Autodesk Inventor part; units mm, degrees
(part 3 of 4)
  spline S47 degree 5 poles (5.1648, 1.4192) (5.1666, 1.4197) (5.1702, 1.4206) (5.1756, 1.4219) (5.1829, 1.4234) (5.1921, 1.425) (5.2013, 1.4263) (5.2105, 1.4276) (5.2198, 1.4287) (5.2291, 1.4298) (5.2384, 1.4308) (5.2477, 1.4317) (5.257, 1.4326) (5.2664, 1.4333) (5.2758, 1.434) (5.2852, 1.4345) (5.2947, 1.435) (5.3041, 1.4354) (5.3136, 1.4357) (5.3231, 1.436) (5.3326, 1.4362) (5.3421, 1.4363) (5.3517, 1.4364) (5.3612, 1.4364) (5.3708, 1.4363) (5.3803, 1.4362) (5.3899, 1.436) (5.3995, 1.4357) (5.4091, 1.4354) (5.4188, 1.4351) (5.4284, 1.4347) (5.4381, 1.4342) (5.4477, 1.4337) (5.4574, 1.4331) (5.4671, 1.4324) (5.4768, 1.4317) (5.4865, 1.431) (5.4962, 1.4302) (5.5059, 1.4294) (5.5156, 1.4285) (5.5254, 1.4275) (5.5351, 1.4265) (5.5449, 1.4255) (5.5546, 1.4244) (5.5644, 1.4232) (5.5742, 1.422) (5.584, 1.4208) (5.5938, 1.4195) (5.6036, 1.4182) (5.6134, 1.4168) (5.6232, 1.4154) (5.633, 1.4139) (5.6429, 1.4124) (5.6527, 1.4108) (5.6626, 1.4092) (5.6724, 1.4075) (5.6823, 1.4058) (5.6922, 1.4041) (5.702, 1.4023) (5.7119, 1.4005) (5.7218, 1.3986) (5.7317, 1.3967) (5.7416, 1.3947) (5.7515, 1.3927) (5.7614, 1.3907) (5.7713, 1.3886) (5.7812, 1.3865) (5.7912, 1.3843) (5.8051, 1.3812) (5.817, 1.3785) (5.8269, 1.3761) (5.8349, 1.3742) (5.8408, 1.3728) knots 0 0 0 0 0 0 0.014286 0.028571 0.042857 0.057143 0.071429 0.085714 0.1 0.114286 0.128571 0.142857 0.157143 0.171429 0.185714 0.2 0.214286 0.228571 0.242857 0.257143 0.271429 0.285714 0.3 0.314286 0.328571 0.342857 0.357143 0.371429 0.385714 0.4 0.414286 0.428571 0.442857 0.457143 0.471429 0.485714 0.5 0.514286 0.528571 0.542857 0.557143 0.571429 0.585714 0.6 0.614286 0.628571 0.642857 0.657143 0.671429 0.685714 0.7 0.714286 0.728571 0.742857 0.757143 0.771429 0.785714 0.8 0.814286 0.828571 0.842857 0.857143 0.871429 0.885714 0.9 0.914286 0.928571 0.942857 0.957143 1 1 1 1 1 1
  line L47 (5.1, 1.4019) -> (5.1648, 1.4192)
  arc A48 (5.1, 1.4019) -> (5.0177, 1.6729) centre (0, 0) ccw
  line L48 (5.0177, 1.6729) -> (5.0811, 1.6946)
  spline S48 degree 5 poles (5.0811, 1.6946) (5.0829, 1.6952) (5.0864, 1.6964) (5.0916, 1.6984) (5.0985, 1.7012) (5.107, 1.705) (5.1154, 1.709) (5.1237, 1.7131) (5.1321, 1.7173) (5.1404, 1.7216) (5.1487, 1.7259) (5.157, 1.7303) (5.1652, 1.7348) (5.1734, 1.7394) (5.1816, 1.7441) (5.1897, 1.7489) (5.1978, 1.7537) (5.2059, 1.7587) (5.2139, 1.7637) (5.222, 1.7687) (5.23, 1.7739) (5.238, 1.7791) (5.2459, 1.7843) (5.2539, 1.7896) (5.2618, 1.795) (5.2697, 1.8004) (5.2775, 1.8059) (5.2854, 1.8115) (5.2932, 1.8171) (5.301, 1.8227) (5.3087, 1.8284) (5.3165, 1.8342) (5.3242, 1.84) (5.3319, 1.8459) (5.3396, 1.8518) (5.3473, 1.8578) (5.3549, 1.8638) (5.3626, 1.8698) (5.3702, 1.8759) (5.3778, 1.8821) (5.3853, 1.8883) (5.3929, 1.8946) (5.4004, 1.9009) (5.4079, 1.9072) (5.4154, 1.9136) (5.4228, 1.92) (5.4303, 1.9265) (5.4377, 1.933) (5.4451, 1.9396) (5.4525, 1.9462) (5.4599, 1.9529) (5.4672, 1.9595) (5.4745, 1.9663) (5.4819, 1.9731) (5.4891, 1.9799) (5.4964, 1.9867) (5.5037, 1.9936) (5.5109, 2.0006) (5.5181, 2.0075) (5.5253, 2.0146) (5.5325, 2.0216) (5.5396, 2.0287) (5.5467, 2.0359) (5.5539, 2.043) (5.561, 2.0502) (5.568, 2.0575) (5.5751, 2.0648) (5.5821, 2.0721) (5.5919, 2.0824) (5.6003, 2.0913) (5.6073, 2.0988) (5.6129, 2.1048) (5.617, 2.1093) knots 0 0 0 0 0 0 0.014286 0.028571 0.042857 0.057143 0.071429 0.085714 0.1 0.114286 0.128571 0.142857 0.157143 0.171429 0.185714 0.2 0.214286 0.228571 0.242857 0.257143 0.271429 0.285714 0.3 0.314286 0.328571 0.342857 0.357143 0.371429 0.385714 0.4 0.414286 0.428571 0.442857 0.457143 0.471429 0.485714 0.5 0.514286 0.528571 0.542857 0.557143 0.571429 0.585714 0.6 0.614286 0.628571 0.642857 0.657143 0.671429 0.685714 0.7 0.714286 0.728571 0.742857 0.757143 0.771429 0.785714 0.8 0.814286 0.828571 0.842857 0.857143 0.871429 0.885714 0.9 0.914286 0.928571 0.942857 0.957143 1 1 1 1 1 1
  arc A49 (5.617, 2.1093) -> (5.5352, 2.3155) centre (0, 0) ccw
  spline S49 degree 5 poles (4.8608, 2.25) (4.8625, 2.2507) (4.8659, 2.2522) (4.871, 2.2544) (4.8779, 2.2571) (4.8867, 2.2601) (4.8956, 2.263) (4.9045, 2.2657) (4.9134, 2.2684) (4.9224, 2.2709) (4.9314, 2.2735) (4.9405, 2.2759) (4.9496, 2.2783) (4.9587, 2.2806) (4.9678, 2.2828) (4.977, 2.2849) (4.9863, 2.2869) (4.9955, 2.2888) (5.0048, 2.2907) (5.0142, 2.2925) (5.0235, 2.2943) (5.0329, 2.296) (5.0422, 2.2976) (5.0517, 2.2992) (5.0611, 2.3007) (5.0706, 2.3022) (5.0801, 2.3036) (5.0896, 2.3049) (5.0991, 2.3062) (5.1087, 2.3074) (5.1182, 2.3086) (5.1278, 2.3097) (5.1374, 2.3108) (5.1471, 2.3118) (5.1567, 2.3128) (5.1664, 2.3137) (5.1761, 2.3145) (5.1858, 2.3153) (5.1955, 2.3161) (5.2053, 2.3168) (5.215, 2.3175) (5.2248, 2.3181) (5.2346, 2.3187) (5.2444, 2.3192) (5.2543, 2.3197) (5.2641, 2.3201) (5.274, 2.3205) (5.2838, 2.3209) (5.2937, 2.3212) (5.3036, 2.3214) (5.3136, 2.3216) (5.3235, 2.3218) (5.3335, 2.3219) (5.3434, 2.322) (5.3534, 2.322) (5.3634, 2.322) (5.3734, 2.3219) (5.3834, 2.3219) (5.3934, 2.3217) (5.4035, 2.3215) (5.4136, 2.3213) (5.4236, 2.3211) (5.4337, 2.3207) (5.4438, 2.3204) (5.4539, 2.32) (5.464, 2.3196) (5.4742, 2.3191) (5.4843, 2.3186) (5.4985, 2.3178) (5.5107, 2.3171) (5.5209, 2.3165) (5.5291, 2.3159) (5.5352, 2.3155) knots 0 0 0 0 0 0 0.014286 0.028571 0.042857 0.057143 0.071429 0.085714 0.1 0.114286 0.128571 0.142857 0.157143 0.171429 0.185714 0.2 0.214286 0.228571 0.242857 0.257143 0.271429 0.285714 0.3 0.314286 0.328571 0.342857 0.357143 0.371429 0.385714 0.4 0.414286 0.428571 0.442857 0.457143 0.471429 0.485714 0.5 0.514286 0.528571 0.542857 0.557143 0.571429 0.585714 0.6 0.614286 0.628571 0.642857 0.657143 0.671429 0.685714 0.7 0.714286 0.728571 0.742857 0.757143 0.771429 0.785714 0.8 0.814286 0.828571 0.842857 0.857143 0.871429 0.885714 0.9 0.914286 0.928571 0.942857 0.957143 1 1 1 1 1 1
  line L49 (4.7997, 2.2222) -> (4.8608, 2.25)
  arc A50 (4.7997, 2.2222) -> (4.6739, 2.476) centre (0, 0) ccw
  line L50 (4.6739, 2.476) -> (4.7329, 2.5078)
  spline S50 degree 5 poles (4.7329, 2.5078) (4.7345, 2.5087) (4.7378, 2.5105) (4.7426, 2.5133) (4.7489, 2.5172) (4.7567, 2.5223) (4.7643, 2.5276) (4.7719, 2.533) (4.7794, 2.5386) (4.7869, 2.5442) (4.7944, 2.5498) (4.8018, 2.5555) (4.8092, 2.5613) (4.8166, 2.5672) (4.8238, 2.5732) (4.8311, 2.5792) (4.8383, 2.5854) (4.8454, 2.5916) (4.8525, 2.5978) (4.8596, 2.6041) (4.8667, 2.6105) (4.8737, 2.6169) (4.8807, 2.6234) (4.8876, 2.63) (4.8946, 2.6366) (4.9014, 2.6432) (4.9083, 2.6499) (4.9151, 2.6567) (4.9219, 2.6635) (4.9287, 2.6704) (4.9354, 2.6773) (4.9421, 2.6842) (4.9488, 2.6912) (4.9554, 2.6983) (4.962, 2.7054) (4.9686, 2.7125) (4.9751, 2.7197) (4.9817, 2.727) (4.9882, 2.7343) (4.9946, 2.7416) (5.0011, 2.749) (5.0075, 2.7564) (5.0139, 2.7638) (5.0202, 2.7713) (5.0266, 2.7788) (5.0329, 2.7864) (5.0391, 2.794) (5.0454, 2.8017) (5.0516, 2.8094) (5.0578, 2.8171) (5.064, 2.8249) (5.0701, 2.8327) (5.0762, 2.8405) (5.0823, 2.8484) (5.0884, 2.8564) (5.0944, 2.8643) (5.1005, 2.8723) (5.1064, 2.8803) (5.1124, 2.8884) (5.1183, 2.8965) (5.1243, 2.9047) (5.1301, 2.9128) (5.136, 2.9211) (5.1418, 2.9293) (5.1477, 2.9376) (5.1534, 2.9459) (5.1592, 2.9542) (5.1649, 2.9626) (5.1729, 2.9744) (5.1797, 2.9846) (5.1854, 2.9931) (5.1899, 2.9999) (5.1932, 3.0051) knots 0 0 0 0 0 0 0.014286 0.028571 0.042857 0.057143 0.071429 0.085714 0.1 0.114286 0.128571 0.142857 0.157143 0.171429 0.185714 0.2 0.214286 0.228571 0.242857 0.257143 0.271429 0.285714 0.3 0.314286 0.328571 0.342857 0.357143 0.371429 0.385714 0.4 0.414286 0.428571 0.442857 0.457143 0.471429 0.485714 0.5 0.514286 0.528571 0.542857 0.557143 0.571429 0.585714 0.6 0.614286 0.628571 0.642857 0.657143 0.671429 0.685714 0.7 0.714286 0.728571 0.742857 0.757143 0.771429 0.785714 0.8 0.814286 0.828571 0.842857 0.857143 0.871429 0.885714 0.9 0.914286 0.928571 0.942857 0.957143 1 1 1 1 1 1
  arc A51 (5.1932, 3.0051) -> (5.0786, 3.1949) centre (0, 0) ccw
  spline S51 degree 5 poles (4.4241, 3.0193) (4.4257, 3.0204) (4.4288, 3.0224) (4.4335, 3.0254) (4.4399, 3.0292) (4.4481, 3.0336) (4.4563, 3.0379) (4.4647, 3.0421) (4.473, 3.0461) (4.4815, 3.0502) (4.49, 3.0542) (4.4985, 3.0581) (4.507, 3.0619) (4.5157, 3.0657) (4.5244, 3.0693) (4.5331, 3.0729) (4.5419, 3.0764) (4.5507, 3.0799) (4.5595, 3.0832) (4.5684, 3.0866) (4.5773, 3.0898) (4.5863, 3.0931) (4.5953, 3.0962) (4.6043, 3.0993) (4.6134, 3.1024) (4.6225, 3.1054) (4.6316, 3.1083) (4.6408, 3.1112) (4.65, 3.114) (4.6592, 3.1168) (4.6684, 3.1195) (4.6777, 3.1222) (4.687, 3.1248) (4.6964, 3.1274) (4.7057, 3.13) (4.7151, 3.1325) (4.7245, 3.1349) (4.734, 3.1373) (4.7435, 3.1397) (4.753, 3.142) (4.7625, 3.1442) (4.772, 3.1465) (4.7816, 3.1486) (4.7912, 3.1508) (4.8008, 3.1529) (4.8104, 3.1549) (4.8201, 3.1569) (4.8298, 3.1589) (4.8395, 3.1608) (4.8492, 3.1627) (4.859, 3.1645) (4.8687, 3.1663) (4.8785, 3.1681) (4.8884, 3.1698) (4.8982, 3.1715) (4.9081, 3.1731) (4.9179, 3.1747) (4.9278, 3.1763) (4.9377, 3.1778) (4.9477, 3.1793) (4.9576, 3.1807) (4.9676, 3.1821) (4.9776, 3.1835) (4.9876, 3.1848) (4.9977, 3.1861) (5.0077, 3.1873) (5.0178, 3.1885) (5.0279, 3.1897) (5.042, 3.1913) (5.0542, 3.1926) (5.0644, 3.1936) (5.0725, 3.1944) (5.0786, 3.1949) knots 0 0 0 0 0 0 0.014286 0.028571 0.042857 0.057143 0.071429 0.085714 0.1 0.114286 0.128571 0.142857 0.157143 0.171429 0.185714 0.2 0.214286 0.228571 0.242857 0.257143 0.271429 0.285714 0.3 0.314286 0.328571 0.342857 0.357143 0.371429 0.385714 0.4 0.414286 0.428571 0.442857 0.457143 0.471429 0.485714 0.5 0.514286 0.528571 0.542857 0.557143 0.571429 0.585714 0.6 0.614286 0.628571 0.642857 0.657143 0.671429 0.685714 0.7 0.714286 0.728571 0.742857 0.757143 0.771429 0.785714 0.8 0.814286 0.828571 0.842857 0.857143 0.871429 0.885714 0.9 0.914286 0.928571 0.942857 0.957143 1 1 1 1 1 1
  line L51 (4.3685, 2.9819) -> (4.4241, 3.0193)
  arc A52 (4.3685, 2.9819) -> (4.2026, 3.2115) centre (0, 0) ccw
  line L52 (4.2026, 3.2115) -> (4.2556, 3.2526)
  spline S52 degree 5 poles (4.2556, 3.2526) (4.257, 3.2538) (4.26, 3.2561) (4.2643, 3.2596) (4.2699, 3.2645) (4.2767, 3.2708) (4.2833, 3.2773) (4.2899, 3.2839) (4.2964, 3.2906) (4.3029, 3.2974) (4.3093, 3.3042) (4.3157, 3.311) (4.3221, 3.3179) (4.3283, 3.325) (4.3345, 3.332) (4.3407, 3.3392) (4.3467, 3.3464) (4.3528, 3.3537) (4.3588, 3.3611) (4.3647, 3.3685) (4.3706, 3.3759) (4.3765, 3.3834) (4.3823, 3.391) (4.3881, 3.3986) (4.3938, 3.4062) (4.3995, 3.4139) (4.4052, 3.4217) (4.4108, 3.4295) (4.4164, 3.4373) (4.4219, 3.4452) (4.4274, 3.4531) (4.4329, 3.4611) (4.4383, 3.4691) (4.4437, 3.4771) (4.449, 3.4852) (4.4544, 3.4934) (4.4596, 3.5015) (4.4649, 3.5097) (4.4701, 3.518) (4.4753, 3.5263) (4.4804, 3.5346) (4.4855, 3.543) (4.4906, 3.5514) (4.4956, 3.5598) (4.5006, 3.5683) (4.5056, 3.5768) (4.5105, 3.5853) (4.5154, 3.5939) (4.5203, 3.6025) (4.5251, 3.6112) (4.53, 3.6199) (4.5347, 3.6286) (4.5395, 3.6373) (4.5442, 3.6461) (4.5489, 3.6549) (4.5535, 3.6638) (4.5581, 3.6726) (4.5627, 3.6816) (4.5673, 3.6905) (4.5718, 3.6995) (4.5763, 3.7085) (4.5807, 3.7175) (4.5852, 3.7266) (4.5896, 3.7357) (4.5939, 3.7448) (4.5983, 3.7539) (4.6026, 3.7631) (4.6069, 3.7723) (4.6128, 3.7853) (4.6178, 3.7964) (4.622, 3.8058) (4.6253, 3.8132) (4.6278, 3.8189) knots 0 0 0 0 0 0 0.014286 0.028571 0.042857 0.057143 0.071429 0.085714 0.1 0.114286 0.128571 0.142857 0.157143 0.171429 0.185714 0.2 0.214286 0.228571 0.242857 0.257143 0.271429 0.285714 0.3 0.314286 0.328571 0.342857 0.357143 0.371429 0.385714 0.4 0.414286 0.428571 0.442857 0.457143 0.471429 0.485714 0.5 0.514286 0.528571 0.542857 0.557143 0.571429 0.585714 0.6 0.614286 0.628571 0.642857 0.657143 0.671429 0.685714 0.7 0.714286 0.728571 0.742857 0.757143 0.771429 0.785714 0.8 0.814286 0.828571 0.842857 0.857143 0.871429 0.885714 0.9 0.914286 0.928571 0.942857 0.957143 1 1 1 1 1 1
  arc A53 (4.6278, 3.8189) -> (4.4835, 3.9873) centre (0, 0) ccw
  spline S53 degree 5 poles (3.8668, 3.7063) (3.8682, 3.7076) (3.8709, 3.7101) (3.8751, 3.7138) (3.8808, 3.7186) (3.8881, 3.7244) (3.8955, 3.73) (3.9031, 3.7354) (3.9107, 3.7408) (3.9183, 3.7462) (3.926, 3.7515) (3.9338, 3.7568) (3.9416, 3.762) (3.9495, 3.7671) (3.9574, 3.7722) (3.9655, 3.7771) (3.9736, 3.782) (3.9817, 3.7869) (3.9899, 3.7917) (3.9981, 3.7964) (4.0063, 3.8011) (4.0147, 3.8058) (4.023, 3.8104) (4.0314, 3.8149) (4.0398, 3.8194) (4.0483, 3.8238) (4.0568, 3.8282) (4.0654, 3.8326) (4.074, 3.8369) (4.0826, 3.8412) (4.0913, 3.8454) (4.1, 3.8496) (4.1088, 3.8537) (4.1176, 3.8578) (4.1264, 3.8618) (4.1352, 3.8658) (4.1441, 3.8698) (4.153, 3.8737) (4.162, 3.8776) (4.171, 3.8814) (4.18, 3.8852) (4.189, 3.889) (4.1981, 3.8927) (4.2072, 3.8964) (4.2164, 3.9001) (4.2255, 3.9037) (4.2347, 3.9072) (4.244, 3.9108) (4.2532, 3.9143) (4.2625, 3.9177) (4.2718, 3.9211) (4.2812, 3.9245) (4.2906, 3.9279) (4.3, 3.9312) (4.3094, 3.9344) (4.3188, 3.9377) (4.3283, 3.9409) (4.3378, 3.944) (4.3474, 3.9472) (4.3569, 3.9503) (4.3665, 3.9533) (4.3761, 3.9563) (4.3858, 3.9593) (4.3954, 3.9623) (4.4051, 3.9652) (4.4148, 3.9681) (4.4246, 3.9709) (4.4343, 3.9737) (4.448, 3.9776) (4.4598, 3.9809) (4.4696, 3.9836) (4.4775, 3.9857) (4.4835, 3.9873) knots 0 0 0 0 0 0 0.014286 0.028571 0.042857 0.057143 0.071429 0.085714 0.1 0.114286 0.128571 0.142857 0.157143 0.171429 0.185714 0.2 0.214286 0.228571 0.242857 0.257143 0.271429 0.285714 0.3 0.314286 0.328571 0.342857 0.357143 0.371429 0.385714 0.4 0.414286 0.428571 0.442857 0.457143 0.471429 0.485714 0.5 0.514286 0.528571 0.542857 0.557143 0.571429 0.585714 0.6 0.614286 0.628571 0.642857 0.657143 0.671429 0.685714 0.7 0.714286 0.728571 0.742857 0.757143 0.771429 0.785714 0.8 0.814286 0.828571 0.842857 0.857143 0.871429 0.885714 0.9 0.914286 0.928571 0.942857 0.957143 1 1 1 1 1 1
  line L53 (3.8181, 3.6603) -> (3.8668, 3.7063)
  arc A54 (3.8181, 3.6603) -> (3.6167, 3.8594) centre (0, 0) ccw
  line L54 (3.6167, 3.8594) -> (3.6622, 3.9087)
  spline S54 degree 5 poles (3.6622, 3.9087) (3.6634, 3.9101) (3.6659, 3.9128) (3.6696, 3.917) (3.6743, 3.9228) (3.68, 3.9301) (3.6855, 3.9376) (3.6908, 3.9452) (3.6962, 3.9529) (3.7015, 3.9606) (3.7067, 3.9684) (3.7119, 3.9762) (3.717, 3.9841) (3.722, 3.992) (3.727, 4) (3.7318, 4.0081) (3.7367, 4.0163) (3.7414, 4.0244) (3.7461, 4.0327) (3.7508, 4.0409) (3.7554, 4.0493) (3.7599, 4.0576) (3.7644, 4.066) (3.7689, 4.0745) (3.7733, 4.083) (3.7776, 4.0915) (3.7819, 4.1001) (3.7862, 4.1087) (3.7904, 4.1173) (3.7945, 4.126) (3.7987, 4.1347) (3.8027, 4.1435) (3.8068, 4.1523) (3.8108, 4.1611) (3.8147, 4.17) (3.8186, 4.1789) (3.8225, 4.1878) (3.8263, 4.1968) (3.8301, 4.2058) (3.8338, 4.2148) (3.8375, 4.2239) (3.8412, 4.2329) (3.8448, 4.2421) (3.8484, 4.2512) (3.8519, 4.2604) (3.8554, 4.2696) (3.8589, 4.2788) (3.8623, 4.2881) (3.8657, 4.2974) (3.869, 4.3067) (3.8724, 4.3161) (3.8756, 4.3255) (3.8789, 4.3349) (3.8821, 4.3443) (3.8852, 4.3538) (3.8884, 4.3633) (3.8915, 4.3728) (3.8945, 4.3823) (3.8975, 4.3919) (3.9005, 4.4015) (3.9035, 4.4111) (3.9064, 4.4208) (3.9093, 4.4304) (3.9121, 4.4401) (3.9149, 4.4499) (3.9177, 4.4596) (3.9204, 4.4694) (3.9231, 4.4792) (3.9269, 4.4929) (3.93, 4.5047) (3.9326, 4.5146) (3.9346, 4.5225) (3.9361, 4.5285) knots 0 0 0 0 0 0 0.014286 0.028571 0.042857 0.057143 0.071429 0.085714 0.1 0.114286 0.128571 0.142857 0.157143 0.171429 0.185714 0.2 0.214286 0.228571 0.242857 0.257143 0.271429 0.285714 0.3 0.314286 0.328571 0.342857 0.357143 0.371429 0.385714 0.4 0.414286 0.428571 0.442857 0.457143 0.471429 0.485714 0.5 0.514286 0.528571 0.542857 0.557143 0.571429 0.585714 0.6 0.614286 0.628571 0.642857 0.657143 0.671429 0.685714 0.7 0.714286 0.728571 0.742857 0.757143 0.771429 0.785714 0.8 0.814286 0.828571 0.842857 0.857143 0.871429 0.885714 0.9 0.914286 0.928571 0.942857 0.957143 1 1 1 1 1 1
  arc A55 (3.9361, 4.5285) -> (3.766, 4.6709) centre (0, 0) ccw
  spline S55 degree 5 poles (3.2041, 4.2922) (3.2052, 4.2937) (3.2075, 4.2967) (3.211, 4.301) (3.2158, 4.3067) (3.222, 4.3135) (3.2285, 4.3203) (3.235, 4.3269) (3.2416, 4.3335) (3.2483, 4.34) (3.255, 4.3466) (3.2618, 4.353) (3.2686, 4.3595) (3.2756, 4.3658) (3.2826, 4.3721) (3.2897, 4.3783) (3.2969, 4.3845) (3.3041, 4.3906) (3.3114, 4.3967) (3.3187, 4.4027) (3.3261, 4.4087) (3.3335, 4.4146) (3.341, 4.4206) (3.3485, 4.4264) (3.3561, 4.4322) (3.3637, 4.438) (3.3714, 4.4438) (3.3791, 4.4495) (3.3869, 4.4551) (3.3947, 4.4608) (3.4026, 4.4663) (3.4105, 4.4719) (3.4184, 4.4774) (3.4264, 4.4829) (3.4345, 4.4883) (3.4425, 4.4937) (3.4506, 4.4991) (3.4588, 4.5045) (3.467, 4.5098) (3.4752, 4.515) (3.4835, 4.5203) (3.4918, 4.5255) (3.5001, 4.5306) (3.5085, 4.5358) (3.5169, 4.5409) (3.5254, 4.5459) (3.5339, 4.551) (3.5424, 4.556) (3.551, 4.5609) (3.5595, 4.5659) (3.5682, 4.5708) (3.5768, 4.5756) (3.5855, 4.5805) (3.5943, 4.5853) (3.603, 4.5901) (3.6118, 4.5948) (3.6206, 4.5995) (3.6295, 4.6042) (3.6384, 4.6089) (3.6473, 4.6135) (3.6563, 4.6181) (3.6652, 4.6227) (3.6743, 4.6272) (3.6833, 4.6317) (3.6924, 4.6362) (3.7015, 4.6406) (3.7106, 4.645) (3.7198, 4.6494) (3.7326, 4.6555) (3.7437, 4.6607) (3.753, 4.6649) (3.7604, 4.6683) (3.766, 4.6709) knots 0 0 0 0 0 0 0.014286 0.028571 0.042857 0.057143 0.071429 0.085714 0.1 0.114286 0.128571 0.142857 0.157143 0.171429 0.185714 0.2 0.214286 0.228571 0.242857 0.257143 0.271429 0.285714 0.3 0.314286 0.328571 0.342857 0.357143 0.371429 0.385714 0.4 0.414286 0.428571 0.442857 0.457143 0.471429 0.485714 0.5 0.514286 0.528571 0.542857 0.557143 0.571429 0.585714 0.6 0.614286 0.628571 0.642857 0.657143 0.671429 0.685714 0.7 0.714286 0.728571 0.742857 0.757143 0.771429 0.785714 0.8 0.814286 0.828571 0.842857 0.857143 0.871429 0.885714 0.9 0.914286 0.928571 0.942857 0.957143 1 1 1 1 1 1
  line L55 (3.1636, 4.2388) -> (3.2041, 4.2922)
  arc A56 (3.1636, 4.2388) -> (2.9321, 4.4021) centre (0, 0) ccw
  line L56 (2.9321, 4.4021) -> (2.9689, 4.4582)
  spline S56 degree 5 poles (2.9689, 4.4582) (2.9699, 4.4597) (2.9719, 4.4628) (2.9748, 4.4676) (2.9785, 4.474) (2.9829, 4.4822) (2.9871, 4.4905) (2.9911, 4.4989) (2.9951, 4.5074) (2.9991, 4.5158) (3.003, 4.5244) (3.0068, 4.5329) (3.0105, 4.5415) (3.0142, 4.5502) (3.0178, 4.5589) (3.0212, 4.5677) (3.0246, 4.5765) (3.028, 4.5854) (3.0313, 4.5943) (3.0345, 4.6032) (3.0377, 4.6121) (3.0408, 4.6211) (3.0438, 4.6302) (3.0468, 4.6392) (3.0498, 4.6483) (3.0527, 4.6575) (3.0555, 4.6666) (3.0583, 4.6758) (3.061, 4.685) (3.0637, 4.6943) (3.0663, 4.7036) (3.0689, 4.7129) (3.0714, 4.7222) (3.0739, 4.7316) (3.0763, 4.741) (3.0787, 4.7504) (3.0811, 4.7598) (3.0833, 4.7693) (3.0856, 4.7788) (3.0878, 4.7883) (3.09, 4.7979) (3.0921, 4.8074) (3.0941, 4.817) (3.0962, 4.8267) (3.0981, 4.8363) (3.1001, 4.846) (3.102, 4.8556) (3.1038, 4.8653) (3.1056, 4.8751) (3.1074, 4.8848) (3.1091, 4.8946) (3.1108, 4.9044) (3.1125, 4.9142) (3.1141, 4.924) (3.1156, 4.9339) (3.1172, 4.9438) (3.1186, 4.9537) (3.1201, 4.9636) (3.1215, 4.9735) (3.1229, 4.9835) (3.1242, 4.9935) (3.1255, 5.0034) (3.1267, 5.0135) (3.1279, 5.0235) (3.1291, 5.0335) (3.1302, 5.0436) (3.1313, 5.0537) (3.1324, 5.0638) (3.1338, 5.078) (3.1349, 5.0901) (3.1358, 5.1003) (3.1365, 5.1085) (3.1371, 5.1146) knots 0 0 0 0 0 0 0.014286 0.028571 0.042857 0.057143 0.071429 0.085714 0.1 0.114286 0.128571 0.142857 0.157143 0.171429 0.185714 0.2 0.214286 0.228571 0.242857 0.257143 0.271429 0.285714 0.3 0.314286 0.328571 0.342857 0.357143 0.371429 0.385714 0.4 0.414286 0.428571 0.442857 0.457143 0.471429 0.485714 0.5 0.514286 0.528571 0.542857 0.557143 0.571429 0.585714 0.6 0.614286 0.628571 0.642857 0.657143 0.671429 0.685714 0.7 0.714286 0.728571 0.742857 0.757143 0.771429 0.785714 0.8 0.814286 0.828571 0.842857 0.857143 0.871429 0.885714 0.9 0.914286 0.928571 0.942857 0.957143 1 1 1 1 1 1
  arc A57 (3.1371, 5.1146) -> (2.9459, 5.227) centre (0, 0) ccw
  spline S57 degree 5 poles (2.4539, 4.7611) (2.4547, 4.7627) (2.4565, 4.766) (2.4592, 4.7709) (2.4631, 4.7772) (2.4681, 4.785) (2.4733, 4.7927) (2.4787, 4.8003) (2.4841, 4.8079) (2.4896, 4.8155) (2.4952, 4.823) (2.5008, 4.8305) (2.5065, 4.838) (2.5123, 4.8454) (2.5182, 4.8528) (2.5242, 4.8601) (2.5302, 4.8673) (2.5364, 4.8745) (2.5425, 4.8817) (2.5488, 4.8889) (2.5551, 4.896) (2.5614, 4.9031) (2.5678, 4.9102) (2.5743, 4.9172) (2.5808, 4.9242) (2.5874, 4.9311) (2.594, 4.9381) (2.6007, 4.945) (2.6074, 4.9518) (2.6142, 4.9587) (2.621, 4.9655) (2.6279, 4.9723) (2.6349, 4.979) (2.6418, 4.9857) (2.6489, 4.9924) (2.6559, 4.9991) (2.6631, 5.0057) (2.6702, 5.0123) (2.6774, 5.0189) (2.6847, 5.0254) (2.692, 5.032) (2.6993, 5.0385) (2.7067, 5.0449) (2.7141, 5.0514) (2.7216, 5.0578) (2.7291, 5.0642) (2.7366, 5.0705) (2.7442, 5.0769) (2.7518, 5.0832) (2.7595, 5.0895) (2.7672, 5.0957) (2.7749, 5.102) (2.7827, 5.1082) (2.7905, 5.1144) (2.7984, 5.1205) (2.8063, 5.1266) (2.8142, 5.1328) (2.8222, 5.1388) (2.8302, 5.1449) (2.8382, 5.1509) (2.8463, 5.1569) (2.8544, 5.1629) (2.8625, 5.1689) (2.8707, 5.1748) (2.8789, 5.1807) (2.8872, 5.1866) (2.8955, 5.1924) (2.9038, 5.1983) (2.9155, 5.2064) (2.9256, 5.2133) (2.934, 5.219) (2.9408, 5.2236) (2.9459, 5.227) knots 0 0 0 0 0 0 0.014286 0.028571 0.042857 0.057143 0.071429 0.085714 0.1 0.114286 0.128571 0.142857 0.157143 0.171429 0.185714 0.2 0.214286 0.228571 0.242857 0.257143 0.271429 0.285714 0.3 0.314286 0.328571 0.342857 0.357143 0.371429 0.385714 0.4 0.414286 0.428571 0.442857 0.457143 0.471429 0.485714 0.5 0.514286 0.528571 0.542857 0.557143 0.571429 0.585714 0.6 0.614286 0.628571 0.642857 0.657143 0.671429 0.685714 0.7 0.714286 0.728571 0.742857 0.757143 0.771429 0.785714 0.8 0.814286 0.828571 0.842857 0.857143 0.871429 0.885714 0.9 0.914286 0.928571 0.942857 0.957143 1 1 1 1 1 1
  line L57 (2.4227, 4.7017) -> (2.4539, 4.7611)
  arc A58 (2.4227, 4.7017) -> (2.1676, 4.8247) centre (0, 0) ccw
  line L58 (2.1676, 4.8247) -> (2.1946, 4.886)
  spline S58 degree 5 poles (2.1946, 4.886) (2.1953, 4.8877) (2.1968, 4.8911) (2.1989, 4.8963) (2.2015, 4.9033) (2.2045, 4.9121) (2.2072, 4.9209) (2.2099, 4.9299) (2.2124, 4.9389) (2.2149, 4.9479) (2.2173, 4.9569) (2.2197, 4.966) (2.222, 4.9751) (2.2241, 4.9843) (2.2262, 4.9935) (2.2282, 5.0027) (2.2301, 5.0119) (2.232, 5.0212) (2.2337, 5.0305) (2.2354, 5.0399) (2.2371, 5.0492) (2.2387, 5.0586) (2.2402, 5.068) (2.2417, 5.0775) (2.2431, 5.0869) (2.2444, 5.0964) (2.2457, 5.1059) (2.2469, 5.1154) (2.2481, 5.125) (2.2492, 5.1345) (2.2503, 5.1441) (2.2513, 5.1537) (2.2523, 5.1634) (2.2532, 5.173) (2.254, 5.1827) (2.2548, 5.1924) (2.2556, 5.2021) (2.2563, 5.2118) (2.2569, 5.2215) (2.2575, 5.2313) (2.2581, 5.241) (2.2586, 5.2508) (2.2591, 5.2606) (2.2595, 5.2704) (2.2599, 5.2803) (2.2602, 5.2901) (2.2605, 5.3) (2.2607, 5.3099) (2.2609, 5.3198) (2.261, 5.3297) (2.2611, 5.3396) (2.2612, 5.3495) (2.2612, 5.3595) (2.2611, 5.3694) (2.2611, 5.3794) (2.2609, 5.3894) (2.2608, 5.3994) (2.2606, 5.4094) (2.2603, 5.4195) (2.26, 5.4295) (2.2597, 5.4396) (2.2593, 5.4496) (2.2589, 5.4597) (2.2584, 5.4698) (2.2579, 5.4799) (2.2574, 5.49) (2.2568, 5.5002) (2.2562, 5.5103) (2.2552, 5.5245) (2.2544, 5.5367) (2.2536, 5.5469) (2.2529, 5.555) (2.2524, 5.5612) knots 0 0 0 0 0 0 0.014286 0.028571 0.042857 0.057143 0.071429 0.085714 0.1 0.114286 0.128571 0.142857 0.157143 0.171429 0.185714 0.2 0.214286 0.228571 0.242857 0.257143 0.271429 0.285714 0.3 0.314286 0.328571 0.342857 0.357143 0.371429 0.385714 0.4 0.414286 0.428571 0.442857 0.457143 0.471429 0.485714 0.5 0.514286 0.528571 0.542857 0.557143 0.571429 0.585714 0.6 0.614286 0.628571 0.642857 0.657143 0.671429 0.685714 0.7 0.714286 0.728571 0.742857 0.757143 0.771429 0.785714 0.8 0.814286 0.828571 0.842857 0.857143 0.871429 0.885714 0.9 0.914286 0.928571 0.942857 0.957143 1 1 1 1 1 1
  arc A59 (2.2524, 5.5612) -> (2.0454, 5.6406) centre (0, 0) ccw
  spline S59 degree 5 poles (1.6368, 5.1) (1.6374, 5.1018) (1.6385, 5.1053) (1.6404, 5.1106) (1.6432, 5.1175) (1.6469, 5.126) (1.6507, 5.1345) (1.6548, 5.1429) (1.6589, 5.1512) (1.6631, 5.1596) (1.6673, 5.1679) (1.6716, 5.1763) (1.676, 5.1846) (1.6805, 5.1928) (1.6851, 5.2011) (1.6898, 5.2092) (1.6946, 5.2174) (1.6994, 5.2255) (1.7043, 5.2336) (1.7093, 5.2417) (1.7144, 5.2498) (1.7194, 5.2578) (1.7246, 5.2658) (1.7298, 5.2738) (1.7351, 5.2818) (1.7404, 5.2898) (1.7458, 5.2977) (1.7513, 5.3056) (1.7568, 5.3135) (1.7624, 5.3213) (1.768, 5.3292) (1.7737, 5.337) (1.7794, 5.3448) (1.7852, 5.3526) (1.791, 5.3603) (1.7969, 5.368) (1.8028, 5.3758) (1.8088, 5.3835) (1.8148, 5.3911) (1.8209, 5.3988) (1.827, 5.4064) (1.8332, 5.414) (1.8394, 5.4216) (1.8457, 5.4292) (1.852, 5.4368) (1.8583, 5.4443) (1.8647, 5.4518) (1.8711, 5.4593) (1.8776, 5.4668) (1.8841, 5.4743) (1.8907, 5.4817) (1.8973, 5.4891) (1.904, 5.4965) (1.9107, 5.5039) (1.9174, 5.5113) (1.9242, 5.5186) (1.931, 5.5259) (1.9378, 5.5333) (1.9447, 5.5405) (1.9517, 5.5478) (1.9587, 5.5551) (1.9657, 5.5623) (1.9727, 5.5695) (1.9798, 5.5767) (1.9869, 5.5839) (1.9941, 5.591) (2.0013, 5.5982) (2.0086, 5.6053) (2.0188, 5.6152) (2.0276, 5.6237) (2.035, 5.6308) (2.0409, 5.6364) (2.0454, 5.6406) knots 0 0 0 0 0 0 0.014286 0.028571 0.042857 0.057143 0.071429 0.085714 0.1 0.114286 0.128571 0.142857 0.157143 0.171429 0.185714 0.2 0.214286 0.228571 0.242857 0.257143 0.271429 0.285714 0.3 0.314286 0.328571 0.342857 0.357143 0.371429 0.385714 0.4 0.414286 0.428571 0.442857 0.457143 0.471429 0.485714 0.5 0.514286 0.528571 0.542857 0.557143 0.571429 0.585714 0.6 0.614286 0.628571 0.642857 0.657143 0.671429 0.685714 0.7 0.714286 0.728571 0.742857 0.757143 0.771429 0.785714 0.8 0.814286 0.828571 0.842857 0.857143 0.871429 0.885714 0.9 0.914286 0.928571 0.942857 0.957143 1 1 1 1 1 1
  line L59 (1.6158, 5.0363) -> (1.6368, 5.1)
  arc A60 (1.6158, 5.0363) -> (1.3439, 5.1156) centre (0, 0) ccw
  line L60 (1.3439, 5.1156) -> (1.3605, 5.1806)
  spline S60 degree 5 poles (1.3605, 5.1806) (1.3609, 5.1824) (1.3618, 5.186) (1.363, 5.1915) (1.3644, 5.1987) (1.3659, 5.2079) (1.3672, 5.2171) (1.3683, 5.2264) (1.3693, 5.2357) (1.3703, 5.245) (1.3712, 5.2543) (1.372, 5.2636) (1.3728, 5.273) (1.3734, 5.2824) (1.374, 5.2918) (1.3744, 5.3012) (1.3748, 5.3106) (1.375, 5.3201) (1.3753, 5.3296) (1.3754, 5.3391) (1.3755, 5.3486) (1.3755, 5.3581) (1.3755, 5.3676) (1.3754, 5.3772) (1.3752, 5.3867) (1.375, 5.3963) (1.3747, 5.4059) (1.3743, 5.4155) (1.3739, 5.4251) (1.3734, 5.4347) (1.3729, 5.4444) (1.3723, 5.454) (1.3717, 5.4636) (1.371, 5.4733) (1.3702, 5.483) (1.3694, 5.4927) (1.3686, 5.5024) (1.3677, 5.5121) (1.3667, 5.5218) (1.3657, 5.5315) (1.3647, 5.5412) (1.3636, 5.551) (1.3624, 5.5607) (1.3612, 5.5705) (1.3599, 5.5802) (1.3586, 5.59) (1.3573, 5.5998) (1.3559, 5.6095) (1.3544, 5.6193) (1.3529, 5.6291) (1.3514, 5.6389) (1.3498, 5.6487) (1.3482, 5.6586) (1.3465, 5.6684) (1.3448, 5.6782) (1.343, 5.688) (1.3412, 5.6979) (1.3394, 5.7077) (1.3375, 5.7176) (1.3355, 5.7275) (1.3335, 5.7373) (1.3315, 5.7472) (1.3294, 5.7571) (1.3273, 5.7669) (1.3252, 5.7768) (1.323, 5.7867) (1.3207, 5.7966) (1.3184, 5.8065) (1.3152, 5.8204) (1.3123, 5.8323) (1.3099, 5.8422) (1.3079, 5.8501) (1.3064, 5.8561) knots 0 0 0 0 0 0 0.014286 0.028571 0.042857 0.057143 0.071429 0.085714 0.1 0.114286 0.128571 0.142857 0.157143 0.171429 0.185714 0.2 0.214286 0.228571 0.242857 0.257143 0.271429 0.285714 0.3 0.314286 0.328571 0.342857 0.357143 0.371429 0.385714 0.4 0.414286 0.428571 0.442857 0.457143 0.471429 0.485714 0.5 0.514286 0.528571 0.542857 0.557143 0.571429 0.585714 0.6 0.614286 0.628571 0.642857 0.657143 0.671429 0.685714 0.7 0.714286 0.728571 0.742857 0.757143 0.771429 0.785714 0.8 0.814286 0.828571 0.842857 0.857143 0.871429 0.885714 0.9 0.914286 0.928571 0.942857 0.957143 1 1 1 1 1 1
  arc A61 (1.3064, 5.8561) -> (1.0891, 5.9003) centre (0, 0) ccw
  spline S61 degree 5 poles (0.775, 5.2999) (0.7753, 5.3017) (0.7759, 5.3054) (0.7769, 5.3109) (0.7785, 5.3181) (0.7807, 5.3272) (0.7831, 5.3361) (0.7857, 5.3451) (0.7884, 5.354) (0.7911, 5.363) (0.7939, 5.3719) (0.7968, 5.3808) (0.7998, 5.3897) (0.8029, 5.3986) (0.8061, 5.4075) (0.8094, 5.4163) (0.8127, 5.4252) (0.8162, 5.434) (0.8197, 5.4428) (0.8232, 5.4516) (0.8269, 5.4604) (0.8306, 5.4691) (0.8343, 5.4779) (0.8382, 5.4866) (0.8421, 5.4954) (0.846, 5.5041) (0.8501, 5.5128) (0.8542, 5.5215) (0.8583, 5.5302) (0.8625, 5.5388) (0.8667, 5.5475) (0.8711, 5.5561) (0.8754, 5.5648) (0.8798, 5.5734) (0.8843, 5.582) (0.8888, 5.5906) (0.8934, 5.5992) (0.898, 5.6078) (0.9027, 5.6163) (0.9075, 5.6249) (0.9122, 5.6334) (0.9171, 5.6419) (0.9219, 5.6504) (0.9269, 5.6589) (0.9318, 5.6674) (0.9369, 5.6759) (0.9419, 5.6844) (0.947, 5.6928) (0.9522, 5.7013) (0.9574, 5.7097) (0.9627, 5.7181) (0.968, 5.7265) (0.9733, 5.7349) (0.9787, 5.7433) (0.9841, 5.7517) (0.9896, 5.7601) (0.9951, 5.7684) (1.0007, 5.7767) (1.0063, 5.7851) (1.0119, 5.7934) (1.0176, 5.8017) (1.0233, 5.81) (1.0291, 5.8183) (1.0349, 5.8265) (1.0408, 5.8348) (1.0467, 5.843) (1.0526, 5.8512) (1.0586, 5.8595) (1.067, 5.8709) (1.0743, 5.8808) (1.0804, 5.8889) (1.0853, 5.8954) (1.0891, 5.9003) knots 0 0 0 0 0 0 0.014286 0.028571 0.042857 0.057143 0.071429 0.085714 0.1 0.114286 0.128571 0.142857 0.157143 0.171429 0.185714 0.2 0.214286 0.228571 0.242857 0.257143 0.271429 0.285714 0.3 0.314286 0.328571 0.342857 0.357143 0.371429 0.385714 0.4 0.414286 0.428571 0.442857 0.457143 0.471429 0.485714 0.5 0.514286 0.528571 0.542857 0.557143 0.571429 0.585714 0.6 0.614286 0.628571 0.642857 0.657143 0.671429 0.685714 0.7 0.714286 0.728571 0.742857 0.757143 0.771429 0.785714 0.8 0.814286 0.828571 0.842857 0.857143 0.871429 0.885714 0.9 0.914286 0.928571 0.942857 0.957143 1 1 1 1 1 1
  line L61 (0.7648, 5.2336) -> (0.775, 5.2999)
  arc A62 (0.7648, 5.2336) -> (0.4836, 5.267) centre (0, 0) ccw
  line L62 (0.4836, 5.267) -> (0.4892, 5.3339)
  spline S62 degree 5 poles (0.4892, 5.3339) (0.4894, 5.3357) (0.4896, 5.3394) (0.4899, 5.345) (0.4901, 5.3524) (0.4901, 5.3617) (0.4898, 5.371) (0.4894, 5.3803) (0.4889, 5.3896) (0.4883, 5.399) (0.4877, 5.4083) (0.487, 5.4177) (0.4862, 5.427) (0.4852, 5.4364) (0.4842, 5.4457) (0.4831, 5.4551) (0.4819, 5.4645) (0.4806, 5.4739) (0.4793, 5.4833) (0.4779, 5.4926) (0.4764, 5.502) (0.4749, 5.5114) (0.4732, 5.5208) (0.4716, 5.5302) (0.4698, 5.5396) (0.468, 5.549) (0.4662, 5.5584) (0.4642, 5.5678) (0.4622, 5.5772) (0.4602, 5.5867) (0.4581, 5.5961) (0.4559, 5.6055) (0.4537, 5.6149) (0.4514, 5.6243) (0.4491, 5.6337) (0.4467, 5.6432) (0.4443, 5.6526) (0.4418, 5.662) (0.4392, 5.6714) (0.4366, 5.6808) (0.434, 5.6903) (0.4313, 5.6997) (0.4286, 5.7091) (0.4258, 5.7185) (0.4229, 5.7279) (0.42, 5.7374) (0.4171, 5.7468) (0.4141, 5.7562) (0.4111, 5.7656) (0.408, 5.775) (0.4048, 5.7845) (0.4017, 5.7939) (0.3984, 5.8033) (0.3952, 5.8127) (0.3918, 5.8221) (0.3885, 5.8315) (0.3851, 5.8409) (0.3816, 5.8503) (0.3781, 5.8598) (0.3746, 5.8692) (0.371, 5.8786) (0.3674, 5.888) (0.3637, 5.8974) (0.36, 5.9068) (0.3563, 5.9161) (0.3525, 5.9255) (0.3486, 5.9349) (0.3447, 5.9443) (0.3392, 5.9575) (0.3345, 5.9687) (0.3304, 5.9781) (0.3272, 5.9856) (0.3247, 5.9912) knots 0 0 0 0 0 0 0.014286 0.028571 0.042857 0.057143 0.071429 0.085714 0.1 0.114286 0.128571 0.142857 0.157143 0.171429 0.185714 0.2 0.214286 0.228571 0.242857 0.257143 0.271429 0.285714 0.3 0.314286 0.328571 0.342857 0.357143 0.371429 0.385714 0.4 0.414286 0.428571 0.442857 0.457143 0.471429 0.485714 0.5 0.514286 0.528571 0.542857 0.557143 0.571429 0.585714 0.6 0.614286 0.628571 0.642857 0.657143 0.671429 0.685714 0.7 0.714286 0.728571 0.742857 0.757143 0.771429 0.785714 0.8 0.814286 0.828571 0.842857 0.857143 0.871429 0.885714 0.9 0.914286 0.928571 0.942857 0.957143 1 1 1 1 1 1
  arc A63 (0.3247, 5.9912) -> (0.103, 5.9991) centre (0, 0) ccw
  spline S63 degree 5 poles (-0.1079, 5.3552) (-0.1079, 5.357) (-0.1079, 5.3607) (-0.1078, 5.3663) (-0.1075, 5.3737) (-0.1068, 5.383) (-0.1059, 5.3922) (-0.1048, 5.4015) (-0.1036, 5.4108) (-0.1024, 5.42) (-0.1011, 5.4293) (-0.0997, 5.4386) (-0.0982, 5.4479) (-0.0966, 5.4571) (-0.095, 5.4664) (-0.0932, 5.4757) (-0.0913, 5.4849) (-0.0894, 5.4942) (-0.0874, 5.5035) (-0.0853, 5.5127) (-0.0831, 5.522) (-0.0809, 5.5312) (-0.0787, 5.5405) (-0.0763, 5.5498) (-0.0739, 5.559) (-0.0714, 5.5683) (-0.0689, 5.5775) (-0.0663, 5.5868) (-0.0636, 5.596) (-0.0609, 5.6052) (-0.0582, 5.6145) (-0.0553, 5.6237) (-0.0525, 5.633) (-0.0495, 5.6422) (-0.0465, 5.6514) (-0.0435, 5.6606) (-0.0404, 5.6699) (-0.0372, 5.6791) (-0.034, 5.6883) (-0.0307, 5.6975) (-0.0274, 5.7067) (-0.0241, 5.7159) (-0.0207, 5.7251) (-0.0172, 5.7343) (-0.0137, 5.7435) (-0.0101, 5.7527) (-0.0065, 5.7619) (-0.0029, 5.7711) (0.0008, 5.7803) (0.0046, 5.7894) (0.0084, 5.7986) (0.0122, 5.8078) (0.0161, 5.8169) (0.02, 5.8261) (0.024, 5.8352) (0.028, 5.8444) (0.0321, 5.8535) (0.0362, 5.8627) (0.0404, 5.8718) (0.0446, 5.8809) (0.0488, 5.8901) (0.0531, 5.8992) (0.0574, 5.9083) (0.0618, 5.9174) (0.0662, 5.9265) (0.0707, 5.9356) (0.0752, 5.9447) (0.0797, 5.9538) (0.0861, 5.9665) (0.0917, 5.9774) (0.0964, 5.9864) (0.1002, 5.9937) (0.103, 5.9991) knots 0 0 0 0 0 0 0.014286 0.028571 0.042857 0.057143 0.071429 0.085714 0.1 0.114286 0.128571 0.142857 0.157143 0.171429 0.185714 0.2 0.214286 0.228571 0.242857 0.257143 0.271429 0.285714 0.3 0.314286 0.328571 0.342857 0.357143 0.371429 0.385714 0.4 0.414286 0.428571 0.442857 0.457143 0.471429 0.485714 0.5 0.514286 0.528571 0.542857 0.557143 0.571429 0.585714 0.6 0.614286 0.628571 0.642857 0.657143 0.671429 0.685714 0.7 0.714286 0.728571 0.742857 0.757143 0.771429 0.785714 0.8 0.814286 0.828571 0.842857 0.857143 0.871429 0.885714 0.9 0.914286 0.928571 0.942857 0.957143 1 1 1 1 1 1
  line L63 (-0.107, 5.2881) -> (-0.1079, 5.3552)
  arc A64 (-0.107, 5.2881) -> (-0.39, 5.2748) centre (0, 0) ccw
  line L64 (-0.39, 5.2748) -> (-0.3954, 5.3416)
  spline S64 degree 5 poles (-0.3954, 5.3416) (-0.3955, 5.3435) (-0.3959, 5.3472) (-0.3965, 5.3527) (-0.3975, 5.3601) (-0.3991, 5.3692) (-0.4009, 5.3784) (-0.4029, 5.3875) (-0.4049, 5.3966) (-0.407, 5.4057) (-0.4092, 5.4148) (-0.4114, 5.4239) (-0.4137, 5.433) (-0.4162, 5.4421) (-0.4187, 5.4512) (-0.4214, 5.4602) (-0.4241, 5.4693) (-0.4269, 5.4783) (-0.4298, 5.4874) (-0.4327, 5.4964) (-0.4357, 5.5054) (-0.4388, 5.5144) (-0.4419, 5.5234) (-0.4451, 5.5324) (-0.4484, 5.5414) (-0.4517, 5.5504) (-0.4551, 5.5593) (-0.4585, 5.5683) (-0.4621, 5.5773) (-0.4656, 5.5862) (-0.4693, 5.5951) (-0.4729, 5.6041) (-0.4767, 5.613) (-0.4805, 5.6219) (-0.4843, 5.6308) (-0.4882, 5.6397) (-0.4922, 5.6486) (-0.4962, 5.6575) (-0.5002, 5.6664) (-0.5044, 5.6752) (-0.5085, 5.6841) (-0.5127, 5.6929) (-0.517, 5.7018) (-0.5213, 5.7106) (-0.5256, 5.7194) (-0.53, 5.7282) (-0.5345, 5.7371) (-0.539, 5.7459) (-0.5435, 5.7546) (-0.5481, 5.7634) (-0.5528, 5.7722) (-0.5575, 5.781) (-0.5622, 5.7897) (-0.567, 5.7985) (-0.5718, 5.8072) (-0.5766, 5.8159) (-0.5816, 5.8247) (-0.5865, 5.8334) (-0.5915, 5.8421) (-0.5965, 5.8508) (-0.6016, 5.8594) (-0.6067, 5.8681) (-0.6119, 5.8768) (-0.6171, 5.8854) (-0.6224, 5.8941) (-0.6277, 5.9027) (-0.633, 5.9114) (-0.6384, 5.92) (-0.646, 5.932) (-0.6525, 5.9424) (-0.658, 5.9509) (-0.6625, 5.9578) (-0.6659, 5.9629) knots 0 0 0 0 0 0 0.014286 0.028571 0.042857 0.057143 0.071429 0.085714 0.1 0.114286 0.128571 0.142857 0.157143 0.171429 0.185714 0.2 0.214286 0.228571 0.242857 0.257143 0.271429 0.285714 0.3 0.314286 0.328571 0.342857 0.357143 0.371429 0.385714 0.4 0.414286 0.428571 0.442857 0.457143 0.471429 0.485714 0.5 0.514286 0.528571 0.542857 0.557143 0.571429 0.585714 0.6 0.614286 0.628571 0.642857 0.657143 0.671429 0.685714 0.7 0.714286 0.728571 0.742857 0.757143 0.771429 0.785714 0.8 0.814286 0.828571 0.842857 0.857143 0.871429 0.885714 0.9 0.914286 0.928571 0.942857 0.957143 1 1 1 1 1 1
  arc A65 (-0.6659, 5.9629) -> (-0.8858, 5.9343) centre (0, 0) ccw
  spline S65 degree 5 poles (-0.9879, 5.2644) (-0.9882, 5.2662) (-0.9888, 5.2699) (-0.9896, 5.2754) (-0.9905, 5.2828) (-0.9913, 5.292) (-0.9919, 5.3013) (-0.9924, 5.3106) (-0.9928, 5.3199) (-0.9931, 5.3293) (-0.9933, 5.3386) (-0.9935, 5.348) (-0.9936, 5.3574) (-0.9935, 5.3668) (-0.9934, 5.3762) (-0.9932, 5.3857) (-0.9929, 5.3951) (-0.9925, 5.4046) (-0.992, 5.414) (-0.9915, 5.4235) (-0.9909, 5.433) (-0.9902, 5.4425) (-0.9895, 5.452) (-0.9887, 5.4615) (-0.9879, 5.471) (-0.987, 5.4806) (-0.986, 5.4901) (-0.985, 5.4997) (-0.9839, 5.5092) (-0.9827, 5.5188) (-0.9815, 5.5283) (-0.9802, 5.5379) (-0.9789, 5.5475) (-0.9775, 5.5571) (-0.9761, 5.5667) (-0.9746, 5.5763) (-0.973, 5.5859) (-0.9715, 5.5955) (-0.9698, 5.6051) (-0.9681, 5.6147) (-0.9664, 5.6244) (-0.9646, 5.634) (-0.9627, 5.6436) (-0.9608, 5.6533) (-0.9589, 5.6629) (-0.9569, 5.6726) (-0.9548, 5.6822) (-0.9527, 5.6919) (-0.9506, 5.7016) (-0.9484, 5.7112) (-0.9462, 5.7209) (-0.9439, 5.7306) (-0.9416, 5.7402) (-0.9392, 5.7499) (-0.9368, 5.7596) (-0.9343, 5.7693) (-0.9318, 5.779) (-0.9293, 5.7887) (-0.9267, 5.7984) (-0.924, 5.8081) (-0.9213, 5.8178) (-0.9186, 5.8275) (-0.9158, 5.8372) (-0.913, 5.8469) (-0.9102, 5.8566) (-0.9073, 5.8663) (-0.9043, 5.876) (-0.9013, 5.8857) (-0.8971, 5.8993) (-0.8934, 5.9109) (-0.8903, 5.9207) (-0.8877, 5.9284) (-0.8858, 5.9343) knots 0 0 0 0 0 0 0.014286 0.028571 0.042857 0.057143 0.071429 0.085714 0.1 0.114286 0.128571 0.142857 0.157143 0.171429 0.185714 0.2 0.214286 0.228571 0.242857 0.257143 0.271429 0.285714 0.3 0.314286 0.328571 0.342857 0.357143 0.371429 0.385714 0.4 0.414286 0.428571 0.442857 0.457143 0.471429 0.485714 0.5 0.514286 0.528571 0.542857 0.557143 0.571429 0.585714 0.6 0.614286 0.628571 0.642857 0.657143 0.671429 0.685714 0.7 0.714286 0.728571 0.742857 0.757143 0.771429 0.785714 0.8 0.814286 0.828571 0.842857 0.857143 0.871429 0.885714 0.9 0.914286 0.928571 0.942857 0.957143 1 1 1 1 1 1
  line L65 (-0.976, 5.1984) -> (-0.9879, 5.2644)
  arc A66 (-0.976, 5.1984) -> (-1.2528, 5.1387) centre (0, 0) ccw
  line L66 (-1.2528, 5.1387) -> (-1.2692, 5.2037)
  spline S66 degree 5 poles (-1.2692, 5.2037) (-1.2697, 5.2055) (-1.2706, 5.2091) (-1.2721, 5.2145) (-1.2744, 5.2216) (-1.2774, 5.2303) (-1.2807, 5.239) (-1.2841, 5.2477) (-1.2876, 5.2563) (-1.2912, 5.265) (-1.2948, 5.2736) (-1.2985, 5.2822) (-1.3023, 5.2908) (-1.3062, 5.2994) (-1.3102, 5.3079) (-1.3143, 5.3164) (-1.3185, 5.3249) (-1.3228, 5.3333) (-1.3271, 5.3418) (-1.3315, 5.3502) (-1.3359, 5.3586) (-1.3404, 5.367) (-1.345, 5.3753) (-1.3496, 5.3837) (-1.3543, 5.392) (-1.3591, 5.4003) (-1.3639, 5.4086) (-1.3688, 5.4169) (-1.3737, 5.4251) (-1.3787, 5.4334) (-1.3838, 5.4416) (-1.3889, 5.4498) (-1.394, 5.458) (-1.3993, 5.4662) (-1.4045, 5.4743) (-1.4098, 5.4824) (-1.4152, 5.4906) (-1.4206, 5.4987) (-1.4261, 5.5067) (-1.4316, 5.5148) (-1.4371, 5.5229) (-1.4428, 5.5309) (-1.4484, 5.5389) (-1.4541, 5.5469) (-1.4599, 5.5549) (-1.4657, 5.5629) (-1.4715, 5.5708) (-1.4774, 5.5788) (-1.4833, 5.5867) (-1.4893, 5.5946) (-1.4953, 5.6025) (-1.5014, 5.6104) (-1.5075, 5.6182) (-1.5136, 5.6261) (-1.5198, 5.6339) (-1.5261, 5.6417) (-1.5323, 5.6495) (-1.5387, 5.6573) (-1.545, 5.665) (-1.5514, 5.6728) (-1.5579, 5.6805) (-1.5643, 5.6882) (-1.5709, 5.6959) (-1.5774, 5.7036) (-1.584, 5.7113) (-1.5907, 5.7189) (-1.5973, 5.7266) (-1.6041, 5.7342) (-1.6135, 5.7448) (-1.6217, 5.7539) (-1.6286, 5.7615) (-1.6341, 5.7675) (-1.6382, 5.772) knots 0 0 0 0 0 0 0.014286 0.028571 0.042857 0.057143 0.071429 0.085714 0.1 0.114286 0.128571 0.142857 0.157143 0.171429 0.185714 0.2 0.214286 0.228571 0.242857 0.257143 0.271429 0.285714 0.3 0.314286 0.328571 0.342857 0.357143 0.371429 0.385714 0.4 0.414286 0.428571 0.442857 0.457143 0.471429 0.485714 0.5 0.514286 0.528571 0.542857 0.557143 0.571429 0.585714 0.6 0.614286 0.628571 0.642857 0.657143 0.671429 0.685714 0.7 0.714286 0.728571 0.742857 0.757143 0.771429 0.785714 0.8 0.814286 0.828571 0.842857 0.857143 0.871429 0.885714 0.9 0.914286 0.928571 0.942857 0.957143 1 1 1 1 1 1
  arc A67 (-1.6382, 5.772) -> (-1.8505, 5.7075) centre (0, 0) ccw
  spline S67 degree 5 poles (-1.8409, 5.03) (-1.8415, 5.0317) (-1.8427, 5.0352) (-1.8444, 5.0405) (-1.8465, 5.0477) (-1.8489, 5.0567) (-1.851, 5.0657) (-1.853, 5.0748) (-1.8549, 5.084) (-1.8567, 5.0931) (-1.8585, 5.1023) (-1.8602, 5.1115) (-1.8618, 5.1208) (-1.8633, 5.1301) (-1.8648, 5.1394) (-1.8661, 5.1487) (-1.8673, 5.1581) (-1.8685, 5.1675) (-1.8696, 5.1769) (-1.8706, 5.1863) (-1.8716, 5.1958) (-1.8725, 5.2053) (-1.8734, 5.2148) (-1.8742, 5.2243) (-1.8749, 5.2338) (-1.8756, 5.2434) (-1.8762, 5.2529) (-1.8767, 5.2625) (-1.8772, 5.2721) (-1.8777, 5.2818) (-1.878, 5.2914) (-1.8784, 5.301) (-1.8786, 5.3107) (-1.8788, 5.3204) (-1.879, 5.3301) (-1.8791, 5.3398) (-1.8792, 5.3495) (-1.8792, 5.3593) (-1.8791, 5.3691) (-1.8791, 5.3788) (-1.8789, 5.3886) (-1.8787, 5.3984) (-1.8785, 5.4082) (-1.8782, 5.418) (-1.8779, 5.4279) (-1.8775, 5.4377) (-1.8771, 5.4476) (-1.8766, 5.4575) (-1.8761, 5.4673) (-1.8755, 5.4772) (-1.8749, 5.4871) (-1.8742, 5.497) (-1.8735, 5.507) (-1.8728, 5.5169) (-1.872, 5.5269) (-1.8712, 5.5368) (-1.8703, 5.5468) (-1.8694, 5.5568) (-1.8684, 5.5668) (-1.8674, 5.5768) (-1.8663, 5.5868) (-1.8652, 5.5968) (-1.8641, 5.6068) (-1.8629, 5.6168) (-1.8617, 5.6269) (-1.8605, 5.6369) (-1.8591, 5.647) (-1.8578, 5.6571) (-1.8559, 5.6712) (-1.8541, 5.6833) (-1.8526, 5.6934) (-1.8514, 5.7015) (-1.8505, 5.7075) knots 0 0 0 0 0 0 0.014286 0.028571 0.042857 0.057143 0.071429 0.085714 0.1 0.114286 0.128571 0.142857 0.157143 0.171429 0.185714 0.2 0.214286 0.228571 0.242857 0.257143 0.271429 0.285714 0.3 0.314286 0.328571 0.342857 0.357143 0.371429 0.385714 0.4 0.414286 0.428571 0.442857 0.457143 0.471429 0.485714 0.5 0.514286 0.528571 0.542857 0.557143 0.571429 0.585714 0.6 0.614286 0.628571 0.642857 0.657143 0.671429 0.685714 0.7 0.714286 0.728571 0.742857 0.757143 0.771429 0.785714 0.8 0.814286 0.828571 0.842857 0.857143 0.871429 0.885714 0.9 0.914286 0.928571 0.942857 0.957143 1 1 1 1 1 1
  line L67 (-1.8183, 4.9668) -> (-1.8409, 5.03)
  arc A68 (-1.8183, 4.9668) -> (-2.0816, 4.8624) centre (0, 0) ccw
  line L68 (-2.0816, 4.8624) -> (-2.1084, 4.9238)
  spline S68 degree 5 poles (-2.1084, 4.9238) (-2.1091, 4.9255) (-2.1107, 4.9289) (-2.113, 4.934) (-2.1164, 4.9406) (-2.1209, 4.9487) (-2.1255, 4.9568) (-2.1303, 4.9648) (-2.1352, 4.9727) (-2.1402, 4.9807) (-2.1452, 4.9886) (-2.1503, 4.9965) (-2.1554, 5.0043) (-2.1607, 5.0121) (-2.166, 5.0199) (-2.1715, 5.0276) (-2.177, 5.0352) (-2.1826, 5.0429) (-2.1882, 5.0505) (-2.1939, 5.0581) (-2.1997, 5.0656) (-2.2055, 5.0732) (-2.2114, 5.0807) (-2.2174, 5.0881) (-2.2234, 5.0956) (-2.2294, 5.103) (-2.2356, 5.1104) (-2.2417, 5.1177) (-2.248, 5.125) (-2.2542, 5.1323) (-2.2606, 5.1396) (-2.267, 5.1469) (-2.2734, 5.1541) (-2.2799, 5.1613) (-2.2864, 5.1685) (-2.293, 5.1756) (-2.2996, 5.1827) (-2.3063, 5.1898) (-2.313, 5.1969) (-2.3198, 5.204) (-2.3266, 5.211) (-2.3334, 5.218) (-2.3403, 5.225) (-2.3473, 5.2319) (-2.3543, 5.2389) (-2.3613, 5.2458) (-2.3684, 5.2527) (-2.3755, 5.2595) (-2.3826, 5.2664) (-2.3898, 5.2732) (-2.3971, 5.28) (-2.4043, 5.2867) (-2.4116, 5.2935) (-2.419, 5.3002) (-2.4264, 5.3069) (-2.4338, 5.3136) (-2.4413, 5.3202) (-2.4488, 5.3269) (-2.4564, 5.3335) (-2.464, 5.3401) (-2.4716, 5.3466) (-2.4792, 5.3532) (-2.4869, 5.3597) (-2.4947, 5.3662) (-2.5025, 5.3727) (-2.5103, 5.3791) (-2.5181, 5.3855) (-2.526, 5.3919) (-2.5371, 5.4009) (-2.5466, 5.4085) (-2.5547, 5.4148) (-2.5611, 5.4199) (-2.5659, 5.4236) knots 0 0 0 0 0 0 0.014286 0.028571 0.042857 0.057143 0.071429 0.085714 0.1 0.114286 0.128571 0.142857 0.157143 0.171429 0.185714 0.2 0.214286 0.228571 0.242857 0.257143 0.271429 0.285714 0.3 0.314286 0.328571 0.342857 0.357143 0.371429 0.385714 0.4 0.414286 0.428571 0.442857 0.457143 0.471429 0.485714 0.5 0.514286 0.528571 0.542857 0.557143 0.571429 0.585714 0.6 0.614286 0.628571 0.642857 0.657143 0.671429 0.685714 0.7 0.714286 0.728571 0.742857 0.757143 0.771429 0.785714 0.8 0.814286 0.828571 0.842857 0.857143 0.871429 0.885714 0.9 0.914286 0.928571 0.942857 0.957143 1 1 1 1 1 1
  arc A69 (-2.5659, 5.4236) -> (-2.7646, 5.3251) centre (0, 0) ccw
  spline S69 degree 5 poles (-2.6437, 4.6584) (-2.6446, 4.66) (-2.6464, 4.6633) (-2.6489, 4.6682) (-2.6522, 4.6749) (-2.6559, 4.6834) (-2.6595, 4.692) (-2.663, 4.7006) (-2.6664, 4.7093) (-2.6697, 4.7181) (-2.6729, 4.7268) (-2.6762, 4.7356) (-2.6793, 4.7445) (-2.6823, 4.7534) (-2.6852, 4.7624) (-2.6881, 4.7714) (-2.6909, 4.7804) (-2.6936, 4.7895) (-2.6962, 4.7986) (-2.6988, 4.8077) (-2.7013, 4.8169) (-2.7038, 4.8261) (-2.7062, 4.8353) (-2.7085, 4.8445) (-2.7108, 4.8538) (-2.713, 4.8631) (-2.7152, 4.8725) (-2.7173, 4.8819) (-2.7194, 4.8912) (-2.7214, 4.9007) (-2.7234, 4.9101) (-2.7253, 4.9196) (-2.7271, 4.9291) (-2.7289, 4.9386) (-2.7307, 4.9481) (-2.7324, 4.9577) (-2.7341, 4.9673) (-2.7357, 4.9769) (-2.7372, 4.9865) (-2.7388, 4.9962) (-2.7402, 5.0059) (-2.7417, 5.0155) (-2.743, 5.0253) (-2.7444, 5.035) (-2.7457, 5.0448) (-2.7469, 5.0545) (-2.7481, 5.0643) (-2.7493, 5.0741) (-2.7504, 5.084) (-2.7514, 5.0938) (-2.7525, 5.1037) (-2.7535, 5.1136) (-2.7544, 5.1235) (-2.7553, 5.1334) (-2.7562, 5.1434) (-2.757, 5.1533) (-2.7577, 5.1633) (-2.7585, 5.1733) (-2.7592, 5.1833) (-2.7598, 5.1933) (-2.7604, 5.2034) (-2.761, 5.2134) (-2.7615, 5.2235) (-2.762, 5.2336) (-2.7625, 5.2437) (-2.7629, 5.2538) (-2.7633, 5.264) (-2.7636, 5.2741) (-2.764, 5.2884) (-2.7643, 5.3006) (-2.7645, 5.3108) (-2.7646, 5.319) (-2.7646, 5.3251) knots 0 0 0 0 0 0 0.014286 0.028571 0.042857 0.057143 0.071429 0.085714 0.1 0.114286 0.128571 0.142857 0.157143 0.171429 0.185714 0.2 0.214286 0.228571 0.242857 0.257143 0.271429 0.285714 0.3 0.314286 0.328571 0.342857 0.357143 0.371429 0.385714 0.4 0.414286 0.428571 0.442857 0.457143 0.471429 0.485714 0.5 0.514286 0.528571 0.542857 0.557143 0.571429 0.585714 0.6 0.614286 0.628571 0.642857 0.657143 0.671429 0.685714 0.7 0.714286 0.728571 0.742857 0.757143 0.771429 0.785714 0.8 0.814286 0.828571 0.842857 0.857143 0.871429 0.885714 0.9 0.914286 0.928571 0.942857 0.957143 1 1 1 1 1 1
  line L69 (-2.611, 4.5998) -> (-2.6437, 4.6584)
  arc A70 (-2.611, 4.5998) -> (-2.8535, 4.4534) centre (0, 0) ccw
  line L70 (-2.8535, 4.4534) -> (-2.8901, 4.5096)
  spline S70 degree 5 poles (-2.8901, 4.5096) (-2.8911, 4.5112) (-2.8932, 4.5143) (-2.8963, 4.5189) (-2.9007, 4.5249) (-2.9065, 4.5322) (-2.9124, 4.5393) (-2.9185, 4.5464) (-2.9246, 4.5534) (-2.9308, 4.5605) (-2.937, 4.5674) (-2.9433, 4.5744) (-2.9497, 4.5813) (-2.9562, 4.5881) (-2.9627, 4.5949) (-2.9694, 4.6016) (-2.9761, 4.6082) (-2.9828, 4.6149) (-2.9897, 4.6214) (-2.9965, 4.628) (-3.0035, 4.6345) (-3.0105, 4.6409) (-3.0175, 4.6474) (-3.0246, 4.6538) (-3.0317, 4.6601) (-3.0389, 4.6664) (-3.0462, 4.6727) (-3.0535, 4.6789) (-3.0609, 4.6851) (-3.0683, 4.6913) (-3.0757, 4.6974) (-3.0832, 4.7035) (-3.0907, 4.7096) (-3.0983, 4.7156) (-3.1059, 4.7216) (-3.1136, 4.7276) (-3.1213, 4.7336) (-3.129, 4.7395) (-3.1368, 4.7453) (-3.1447, 4.7512) (-3.1525, 4.757) (-3.1605, 4.7628) (-3.1684, 4.7685) (-3.1764, 4.7742) (-3.1844, 4.7799) (-3.1925, 4.7856) (-3.2006, 4.7912) (-3.2088, 4.7968) (-3.2169, 4.8024) (-3.2252, 4.8079) (-3.2334, 4.8134) (-3.2417, 4.8189) (-3.25, 4.8243) (-3.2584, 4.8298) (-3.2668, 4.8351) (-3.2752, 4.8405) (-3.2837, 4.8458) (-3.2922, 4.8511) (-3.3007, 4.8564) (-3.3093, 4.8617) (-3.3179, 4.8669) (-3.3265, 4.8721) (-3.3352, 4.8772) (-3.3439, 4.8824) (-3.3526, 4.8875) (-3.3614, 4.8926) (-3.3702, 4.8976) (-3.379, 4.9026) (-3.3914, 4.9096) (-3.4021, 4.9156) (-3.4111, 4.9205) (-3.4183, 4.9244) (-3.4237, 4.9273) knots 0 0 0 0 0 0 0.014286 0.028571 0.042857 0.057143 0.071429 0.085714 0.1 0.114286 0.128571 0.142857 0.157143 0.171429 0.185714 0.2 0.214286 0.228571 0.242857 0.257143 0.271429 0.285714 0.3 0.314286 0.328571 0.342857 0.357143 0.371429 0.385714 0.4 0.414286 0.428571 0.442857 0.457143 0.471429 0.485714 0.5 0.514286 0.528571 0.542857 0.557143 0.571429 0.585714 0.6 0.614286 0.628571 0.642857 0.657143 0.671429 0.685714 0.7 0.714286 0.728571 0.742857 0.757143 0.771429 0.785714 0.8 0.814286 0.828571 0.842857 0.857143 0.871429 0.885714 0.9 0.914286 0.928571 0.942857 0.957143 1 1 1 1 1 1
  arc A71 (-3.4237, 4.9273) -> (-3.6034, 4.7974) centre (0, 0) ccw
  spline S71 degree 5 poles (-3.3744, 4.1597) (-3.3755, 4.1612) (-3.3778, 4.1641) (-3.3812, 4.1685) (-3.3855, 4.1746) (-3.3906, 4.1824) (-3.3955, 4.1902) (-3.4004, 4.1982) (-3.4051, 4.2062) (-3.4098, 4.2143) (-3.4145, 4.2224) (-3.4191, 4.2306) (-3.4237, 4.2388) (-3.4281, 4.2471) (-3.4325, 4.2554) (-3.4368, 4.2638) (-3.441, 4.2723) (-3.4451, 4.2808) (-3.4492, 4.2894) (-3.4533, 4.2979) (-3.4573, 4.3066) (-3.4612, 4.3152) (-3.4651, 4.3239) (-3.469, 4.3327) (-3.4727, 4.3414) (-3.4765, 4.3503) (-3.4802, 4.3591) (-3.4838, 4.368) (-3.4874, 4.3769) (-3.4909, 4.3859) (-3.4944, 4.3949) (-3.4978, 4.4039) (-3.5012, 4.413) (-3.5046, 4.4221) (-3.5079, 4.4312) (-3.5111, 4.4403) (-3.5144, 4.4495) (-3.5175, 4.4587) (-3.5207, 4.468) (-3.5237, 4.4773) (-3.5268, 4.4866) (-3.5298, 4.4959) (-3.5328, 4.5052) (-3.5357, 4.5146) (-3.5386, 4.524) (-3.5414, 4.5335) (-3.5442, 4.5429) (-3.5469, 4.5524) (-3.5497, 4.5619) (-3.5523, 4.5715) (-3.555, 4.581) (-3.5576, 4.5906) (-3.5601, 4.6003) (-3.5627, 4.6099) (-3.5651, 4.6196) (-3.5676, 4.6293) (-3.57, 4.639) (-3.5724, 4.6487) (-3.5747, 4.6585) (-3.577, 4.6682) (-3.5792, 4.6781) (-3.5815, 4.6879) (-3.5836, 4.6977) (-3.5858, 4.7076) (-3.5879, 4.7175) (-3.59, 4.7274) (-3.592, 4.7374) (-3.594, 4.7473) (-3.5967, 4.7613) (-3.599, 4.7733) (-3.6009, 4.7833) (-3.6023, 4.7914) (-3.6034, 4.7974) knots 0 0 0 0 0 0 0.014286 0.028571 0.042857 0.057143 0.071429 0.085714 0.1 0.114286 0.128571 0.142857 0.157143 0.171429 0.185714 0.2 0.214286 0.228571 0.242857 0.257143 0.271429 0.285714 0.3 0.314286 0.328571 0.342857 0.357143 0.371429 0.385714 0.4 0.414286 0.428571 0.442857 0.457143 0.471429 0.485714 0.5 0.514286 0.528571 0.542857 0.557143 0.571429 0.585714 0.6 0.614286 0.628571 0.642857 0.657143 0.671429 0.685714 0.7 0.714286 0.728571 0.742857 0.757143 0.771429 0.785714 0.8 0.814286 0.828571 0.842857 0.857143 0.871429 0.885714 0.9 0.914286 0.928571 0.942857 0.957143 1 1 1 1 1 1
  line L71 (-3.3325, 4.1073) -> (-3.3744, 4.1597)
  arc A72 (-3.3325, 4.1073) -> (-3.5476, 3.923) centre (0, 0) ccw
  line L72 (-3.5476, 3.923) -> (-3.5929, 3.9724)